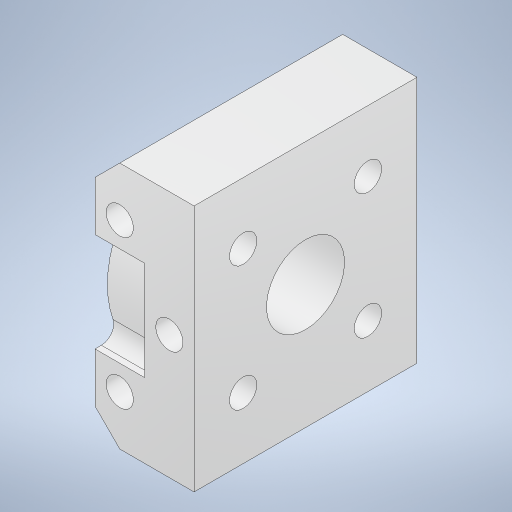
# Autodesk Inventor part: Bracket
Saved by Autodesk Inventor 2023.2 (Build 272271000, 271)
## iProperties
Created: 2024-01-11
Part Number: Bracket
Material: Aluminum 6061
Document SubType Name: Modeling
Designer: Nathan Cai
Mass: 20.3859 g
Surface Area: 41.6637 cm^2
Volume: 7.55035 cm^3
Density: 2.7 g/cm^3
Appearance: Aluminum - Flat
Author: Nathan Cai
Autodesk Inventor part; units mm, degrees
ref_plane "YZ Plane" through (0, 0, 0) normal (1, 0, 0) x (0, 1, 0)
ref_plane "XZ Plane" through (0, 0, 0) normal (0, 1, 0) x (-1, 0, 0)
ref_plane "XY Plane" through (0, 0, 0) normal (0, 0, 1) x (1, 0, 0)
sketch "Sketch1" plane through (0, 0, 0) normal (1, 0, 0) x (0, 1, 0)
  line L0 (-15.875, 14.2875) -> (15.875, 14.2875)
  line L1 (15.875, 14.2875) -> (15.875, -14.2875)
  line L2 (15.875, -14.2875) -> (-15.875, -14.2875)
  line L3 (-15.875, -14.2875) -> (-15.875, 14.2875)
  line L4 (-15.875, 14.2875) -> (15.875, -14.2875) construction
  line L5 (15.875, 14.2875) -> (-15.875, -14.2875) construction
  line L6 (-10, 10) -> (10, 10) construction
  line L7 (10, 10) -> (10, -10) construction
  line L8 (10, -10) -> (-10, -10) construction
  line L9 (-10, -10) -> (-10, 10) construction
  line L10 (-10, 10) -> (10, -10) construction
  line L11 (10, 10) -> (-10, -10) construction
  circle A0 centre (10, 10) radius 1.7526
  circle A1 centre (-10, 10) radius 1.7526
  circle A2 centre (-10, -10) radius 1.7526
  circle A3 centre (10, -10) radius 1.7526
  circle A4 centre (0, 0) radius 17.4625
  circle A5 centre (0, 0) radius 5
  point P0 (-15.875, 7.2748)
  point P1 (-15.875, -7.2748)
  point P2 (15.875, -7.2748)
  point P3 (15.875, 7.2748)
  dimension "d0" = 31.75
  dimension "d1" = 28.575
  dimension "d2" = 20
  dimension "d3" = 20
  dimension "d4" = 3.5052
  dimension "d7" = 360
  dimension "d9" = 34.925
  dimension "d10" = 10
  constraints: 24 end point, 6 centre point, 5 coincident, 4 midpoint, 4 parallel, 2 horizontal, 2 perpendicular, 11 other
  measures "d0" distance of L1.end L2.end
  measures "d1" distance of L0.end L1.end
  measures "d2" distance of L7.end L8.end
  measures "d3" distance of L6.end L7.end
  measures "d4" diameter of A0
  measures "d9" diameter of A4
  measures "d10" diameter of A5
extrude "Extrusion1" add sketch "Sketch1" along normal blind 6.35 contours L0 A4 L3 | L0 A4 L1 L2 L3 | L0 L1 A4 | A4 L2 L3 | L1 L2 A4 | A0 | A1 | A2 | A3
sketch "Sketch3" plane through (0, 0, 0) normal (-1, 0, 0) x (0, 0, 1)
  circle A0 centre (0, 0) radius 12.7
  line L0 (-14.2875, 15.875) -> (14.2875, 15.875) projected
  line L1 (14.2875, 15.875) -> (14.2875, -15.875) projected
  line L2 (-14.2875, 15.875) -> (14.2875, 15.875)
  line L3 (14.2875, 15.875) -> (14.2875, 6.35)
  line L4 (14.2875, 6.35) -> (-14.2875, 6.35)
  line L5 (-14.2875, 6.35) -> (-14.2875, 15.875)
  line L6 (-14.2875, -15.875) -> (-14.2875, 15.875) projected
  line L7 (14.2875, -15.875) -> (-14.2875, -15.875)
  line L8 (-14.2875, -15.875) -> (-14.2875, -6.35)
  line L9 (-14.2875, -6.35) -> (14.2875, -6.35)
  line L10 (14.2875, -6.35) -> (14.2875, -15.875)
  line L11 (14.2875, -15.875) -> (-14.2875, -15.875) projected
  line L12 (14.2875, 15.875) -> (14.2875, -15.875) projected
  line L13 (-14.2875, 15.875) -> (14.2875, 15.875) projected
  line L14 (-14.2875, -15.875) -> (-14.2875, 15.875) projected
  circle A1 centre (0, 0) radius 5 projected
  line L15 (14.2875, -15.875) -> (-14.2875, -15.875) projected
  point P0 (-10.9985, 6.35)
  point P1 (-10.9985, -6.35)
  point P2 (-14.2875, -15.875)
  point P3 (14.2875, -6.35)
  point P4 (10.9985, -6.35)
  point P5 (10.9985, 6.35)
  dimension "d69" = 9.525
  dimension "d70" = 25.4
  dimension "d71" = 9.525
  constraints: 16 end point, 4 parallel, 2 horizontal, 2 perpendicular, 2 point on line, 1 centre point, 1 coincident
  measures "d69" distance between parallel lines of L4 L0
  measures "d70" diameter of A0
  measures "d71" distance between parallel lines of L15 L9
extrude "Extrusion3" add sketch "Sketch3" along normal blind 6.35 contours A0 L9 L4 | L4 A0 | A0 L4 L5 L0 L1 | L9 L1 L7 L6 A0 | A0 L9
fillet "Fillet3" radius 1.5875 4 edges at (-3.175, -6.35, 10.9985) (-3.175, 6.35, 10.9985) (-3.175, -6.35, -10.9985) (-3.175, 6.35, -10.9985)
sketch "Sketch4" plane through (6.35, -15.875, -14.2875) normal (0, 0, -1) x (-1, 0, 0)
  line L0 (12.7, 31.75) -> (12.7, 22.225) projected
  line L1 (12.5475, 25.4) -> (0, 25.4) construction
  line L2 (0, 0) -> (0, 31.75) projected
  line L3 (6.35, 15.875) -> (0, 15.875) construction
  line L4 (6.35, 22.225) -> (12.7, 22.225) projected
  line L5 (9.525, 22.225) -> (9.525, 28.575) construction
  line L6 (12.7, 28.575) -> (0, 28.575) projected
  circle A0 centre (3.175, 15.875) radius 1.75
  line L7 (12.5475, 6.35) -> (0, 6.35) construction
  line L8 (9.525, 9.525) -> (9.525, 3.175) construction
  circle A1 centre (9.525, 25.4) radius 1.75
  circle A2 centre (9.525, 6.35) radius 1.75
  dimension "d37" = 3.5
  dimension "d44" = 9.525
  dimension "d46" = 3.5
  constraints: 10 end point, 5 symmetric about line, 4 midpoint, 3 centre point, 2 point on line, 1 horizontal, 1 vertical, 3 other
  measures "d37" diameter of A0
  measures "d44" distance between parallel lines of L1 L3
  measures "d46" diameter of A1
extrude "Extrusion4" cut sketch "Sketch4" against normal blind 6
chamfer "Chamfer4" distance 1.75 angle 45 3 edges at (4.925, 0, -8.2875) (-1.425, 9.525, -8.2875) (-1.425, -9.525, -8.2875)
mirror "Mirror1" about plane through (0, 0, 0) normal (0, 0, 1) of "Extrusion4", "Chamfer4"
sketch "Sketch5" plane through (-6.35, 0, 0) normal (-1, 0, 0) x (0, 0, 1)
  line L0 (-8, -8) -> (8, -8) construction
  line L1 (8, -8) -> (8, 8) construction
  line L2 (8, 8) -> (-8, 8) construction
  line L3 (-8, 8) -> (-8, -8) construction
  line L4 (-8, -8) -> (8, 8) construction
  line L5 (8, -8) -> (-8, 8) construction
  circle A0 centre (-8, 8) radius 1.7526
  circle A1 centre (-8, -8) radius 1.7526
  circle A2 centre (8, -8) radius 1.7526
  circle A3 centre (8, 8) radius 1.7526
  point P0 (0, 0)
  dimension "d47" = 16
  dimension "d48" = 16
  dimension "d49" = 3.5052
  dimension "d52" = 360
  constraints: 12 end point, 4 centre point, 2 midpoint, 2 parallel, 1 coincident, 1 horizontal, 1 perpendicular, 9 other
  measures "d47" distance of L2.end L1.end
  measures "d48" distance of L1.end L0.end
  measures "d49" diameter of A0
extrude "Extrusion5" cut sketch "Sketch5" against normal through all
sketch "Sketch6" plane through (-6.35, 0, 0) normal (-1, 0, 0) x (0, 0, 1)
  circle A0 centre (0, 0) radius 8
  dimension "d59" = 16
  constraints: 1 centre point, 1 coincident
  measures "d59" diameter of A0
extrude "Extrusion6" cut sketch "Sketch6" against normal blind 5
sketch "Sketch7" plane through (-6.35, 0, 0) normal (-1, 0, 0) x (0, 0, 1)
  circle A0 centre (0, 0) radius 9
  dimension "d62" = 18
  constraints: 1 centre point, 1 coincident
  measures "d62" diameter of A0
extrude "Extrusion7" cut sketch "Sketch7" against normal blind 1
sketch "Sketch9" plane through (-6.35, 0, 0) normal (-1, 0, 0) x (0, 0, 1)
  circle A0 centre (-8, 8) radius 1.7526 projected
  circle A1 centre (-8, 8) radius 3.5719
  circle A2 centre (-8, -8) radius 3.5719
  circle A3 centre (8, -8) radius 3.5719
  circle A4 centre (8, 8) radius 3.5719
  point P0 (0, 0)
  dimension "d72" = 7.1437
  dimension "d75" = 360
  constraints: 4 centre point, 1 coincident, 9 other
  measures "d72" diameter of A1
extrude "Extrusion8" cut sketch "Sketch9" against normal up to surface (1 mm away) contours A0 | A1 | A2 | A3 | A4
fillet "Fillet4" radius 0.7937 8 edges at (-5.85, 7.8331, -4.432) (-5.85, 4.432, -7.8331) (-5.85, 7.8331, 4.432) (-5.85, 4.432, 7.8331) (-5.85, -4.432, 7.8331) (-5.85, -7.8331, 4.432) (-5.85, -7.8331, -4.432) (-5.85, -4.432, -7.8331)
chamfer "Chamfer6" distance 1.5875 angle 49 4 edges at (-5.35, -8, -9.7526) (-5.35, 8, -9.7526) (-5.35, 8, 6.2474) (-5.35, -8, 6.2474) measured on face at (-5.35, 8, -10.2526) measured on face at (-5.35, -8, -10.2526) measured on face at (-5.35, 8, 5.7474) measured on face at (-5.35, -8, 5.7474)
chamfer "Chamfer7" distance 3.175 angle 45 2 edges at (-6.35, 15.875, 0) (-6.35, -15.875, 0)
equation "\"d71\" = d69"
body "Solid1"
